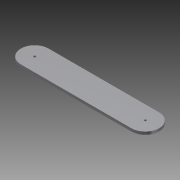
# Autodesk Inventor part: outer drive side
Saved by Autodesk Inventor 2011 (Build 150239000, 239)
## iProperties
Created: 2010-04-20
Part Number: outer drive side
Document SubType Name: Modeling
Designer: lucio
Density: 1 g/cm^3
Mass: 218.635 g
Surface Area: 537.994 cm^2
Volume: 218.635 cm^3
Author: lucio
Autodesk Inventor part; units mm, degrees
ref_plane "YZ Plane" through (0, 0, 0) normal (1, 0, 0) x (0, 1, 0)
ref_plane "XZ Plane" through (0, 0, 0) normal (0, 1, 0) x (-1, 0, 0)
ref_plane "XY Plane" through (0, 0, 0) normal (0, 0, 1) x (1, 0, 0)
sketch "Sketch1" plane through (0, 0, 0) normal (0, 0, 1) x (1, 0, 0)
  line L0 (-419.6966, 0.5698) -> (-19.6966, 0.5698)
  line L1 (-19.6966, 0.5698) -> (-19.6966, 100.5698)
  line L2 (-19.6966, 100.5698) -> (-419.6966, 100.5698)
  line L3 (-419.6966, 100.5698) -> (-419.6966, 0.5698)
  circle A0 centre (-419.6966, 50.5698) radius 50
  circle A1 centre (-19.6966, 50.5698) radius 50
  dimension "d12" = 400
  dimension "d13" = 100
  dimension "d14" = 100
  dimension "d15" = 100
  constraints: 8 end point, 2 centre point, 2 midpoint, 2 parallel, 1 horizontal, 1 perpendicular
  measures "d12" distance of L2.end L1.end
  measures "d13" distance of L1.end L0.end
  measures "d14" diameter of A0
  measures "d15" diameter of A1
extrude "Extrusion1" add sketch "Sketch1" along normal blind 10
sketch "Sketch2" plane through (0, 0, 10) normal (0, 0, 1) x (1, 0, 0)
  arc A0 (-419.6966, 100.5698) -> (-419.6966, 0.5698) centre (-419.6966, 50.5698) ccw projected
  arc A1 (-19.6966, 0.5698) -> (-19.6966, 100.5698) centre (-19.6966, 50.5698) ccw projected
  point P0 (0, 0)
  constraints: 2 coincident
hole "Hole1" at (-419.6966, 50.5698, 10) at (-19.6966, 50.5698, 10) direction (0, 0, -1) diameter 8 end through all
equation "\"d14\" = d13"
equation "\"d15\" = d13"
body "Solid1"
